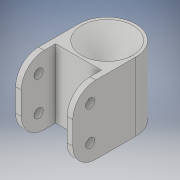
# Autodesk Inventor part: climb pull point
Saved by Autodesk Inventor 2017 SP1 (Build 210196100, 196)
## iProperties
Created: 2018-03-18
Part Number: climb pull point
Material: Generic
Document SubType Name: Modeling
Designer: Ben
Density: 1 g/cm^3
Appearance: Default
Author: Ben
Autodesk Inventor part; units mm, degrees
ref_plane "YZ Plane" through (0, 0, 0) normal (1, 0, 0) x (0, 1, 0)
ref_plane "XZ Plane" through (0, 0, 0) normal (0, 1, 0) x (-1, 0, 0)
ref_plane "XY Plane" through (0, 0, 0) normal (0, 0, 1) x (1, 0, 0)
sketch "Sketch1" plane through (0, 0, 0) normal (0, 1, 0) x (-1, 0, 0)
  line L0 (-15.875, 15.875) -> (15.875, 15.875)
  line L1 (15.875, 15.875) -> (15.875, -15.875)
  line L2 (15.875, -15.875) -> (-15.875, -15.875)
  line L3 (-15.875, -15.875) -> (-15.875, 15.875)
  line L4 (-15.875, 15.875) -> (15.875, -15.875) construction
  line L5 (15.875, 15.875) -> (-15.875, -15.875) construction
  line L6 (-15.875, 15.875) -> (-12.7, 15.875)
  line L7 (-12.7, 15.875) -> (-12.7, 34.925)
  line L8 (-12.7, 34.925) -> (-15.875, 34.925)
  line L9 (-15.875, 34.925) -> (-15.875, 15.875)
  line L10 (15.875, 15.875) -> (12.7, 15.875)
  line L11 (12.7, 15.875) -> (12.7, 34.925)
  line L12 (12.7, 34.925) -> (15.875, 34.925)
  line L13 (15.875, 34.925) -> (15.875, 15.875)
  point P0 (0, 0)
  dimension "d0" = 31.75
  dimension "d13" = 25.4
  dimension "d14" = 19.05
  constraints: 28 end point, 6 parallel, 3 horizontal, 3 perpendicular, 2 equal length, 2 midpoint, 1 point on line
  measures "d0" distance of L1.end L2.end
  measures "d13" distance between parallel lines of L11 L7
  measures "d14" distance of L8.end L0.start
extrude "Extrusion1" add sketch "Sketch1" along normal mid plane 38.1
sketch "Sketch2" plane through (0, 0, 0) normal (0, 1, 0) x (-1, 0, 0)
  circle A0 centre (0, 0) radius 3.175
  dimension "d3" = 6.35
  constraints: 1 centre point, 1 coincident
  measures "d3" diameter of A0
sketch "Sketch3" plane through (0, 19.05, 0) normal (0, 1, 0) x (1, 0, 0)
  circle A0 centre (0, 0) radius 14.2875
  dimension "d4" = 28.575
  constraints: 1 centre point, 1 coincident
  measures "d4" diameter of A0
sketch "Sketch4" plane through (0, -19.05, 0) normal (0, -1, 0) x (1, 0, 0)
  circle A0 centre (0, 0) radius 14.2875
  dimension "d5" = 28.575
  constraints: 1 centre point, 1 coincident
  measures "d5" diameter of A0
loft "Loft1" cut profiles "Sketch3", "Sketch2", "Sketch4"
fillet "Fillet1" radius 15.875 2 edges at (15.875, 0, -15.875) (-15.875, 0, -15.875)
fillet "Fillet1" radius 12.7 4 edges at (14.2875, 19.05, 34.925) (14.2875, -19.05, 34.925) (-14.2875, 19.05, 34.925) (-14.2875, -19.05, 34.925)
sketch "Sketch5" plane through (-15.875, -19.05, 0) normal (-1, 0, 0) x (0, 0, 1)
  line L0 (15.875, 0) -> (15.875, 38.1) construction
  line L1 (15.875, 0) -> (15.875, 38.1) construction
  circle A0 centre (25.4, 9.525) radius 2.54
  circle A1 centre (25.4, 28.575) radius 2.54
  line L2 (25.4, 9.525) -> (25.4, 28.575) construction
  line L3 (25.4, 19.05) -> (0, 19.05) construction
  dimension "d16" = 5.08
  dimension "d17" = 9.525
  dimension "d18" = 19.05
  constraints: 4 end point, 2 centre point, 1 equal radius, 1 horizontal, 1 midpoint, 1 vertical
  measures "d16" diameter of A0
  measures "d17" distance between parallel lines of L0 L2
  measures "d18" distance of L2.start L2.end
extrude "Extrusion2" cut sketch "Sketch5" against normal through all
body "Solid1"
